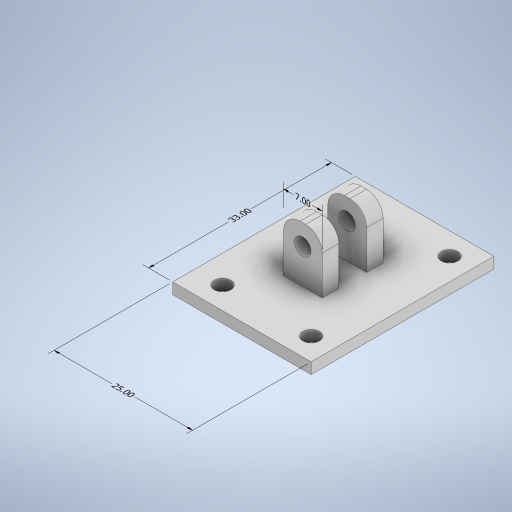
# Autodesk Inventor part: CamBracket
Saved by Autodesk Inventor 2024 (Build 280153000, 153)
## iProperties
Created: 2023-05-15
Part Number: CamBracket
Material: Generic
Document SubType Name: Modeling
Designer: User
Density: 1 g/cm^3
Appearance: Default
Author: User
Autodesk Inventor part; units mm, degrees
ref_plane "YZ Plane" through (0, 0, 0) normal (1, 0, 0) x (0, 1, 0)
ref_plane "XZ Plane" through (0, 0, 0) normal (0, 1, 0) x (-1, 0, 0)
ref_plane "XY Plane" through (0, 0, 0) normal (0, 0, 1) x (1, 0, 0)
sketch "Sketch3" plane through (0, 0, 0) normal (0, 1, 0) x (-1, 0, 0)
  line L0 (0, 0) -> (25, 0)
  line L1 (25, 0) -> (25, -33)
  line L2 (25, -33) -> (0, -33)
  line L3 (0, -33) -> (0, 0)
  dimension "d6" = 25
  dimension "d7" = 33
  constraints: 8 end point, 2 parallel, 1 horizontal, 1 perpendicular
  measures "d6" distance of L1.end L2.end
  measures "d7" distance of L0.end L1.end
extrude "Extrusion2" add sketch "Sketch3" along normal blind 2
sketch "Sketch4" plane through (0, 2, 0) normal (0, 1, 0) x (1, 0, 0)
  circle A0 centre (-4, 4) radius 1.5
  line L0 (0, 0) -> (0, 33) projected
  line L1 (-25, 0) -> (0, 0) projected
  circle A1 centre (-4, 29) radius 1.5
  line L2 (0, 33) -> (-25, 33) projected
  circle A2 centre (-20, 4) radius 1.5
  line L3 (-25, 33) -> (-25, 0) projected
  circle A3 centre (-20, 29) radius 1.5
  dimension "d16" = 3
  dimension "d17" = 4
  dimension "d18" = 4
  dimension "d19" = 3
  dimension "d20" = 4
  dimension "d21" = 4
  dimension "d22" = 3
  dimension "d23" = 16
  dimension "d24" = 4
  dimension "d25" = 5
  dimension "d26" = 3
  dimension "d27" = 4
  dimension "d28" = 16
  dimension "d29" = 25
  constraints: 4 centre point
  measures "d16" diameter of A0
  measures "d17" distance from line of L0 A0.centre
  measures "d18" distance from line of L1 A0.centre
  measures "d19" diameter of A1
  measures "d20" distance from line of L0 A1.centre
  measures "d21" distance from line of L2 A1.centre
  measures "d22" diameter of A2
  measures "d23" distance of A0.centre A2.centre
  measures "d24" distance from line of L1 A2.centre
  measures "d25" distance from line of L3 A2.centre
  measures "d26" diameter of A3
  measures "d27" distance from line of L2 A3.centre
  measures "d28" distance of A1.centre A3.centre
  measures "d29" distance of A1.centre A0.centre
extrude "Extrusion3" cut sketch "Sketch4" against normal blind 2 contours A0 | A1 | A2 | A3
sketch "Sketch5" plane through (0, 2, 0) normal (0, 1, 0) x (1, 0, 0)
  line L0 (-16, 11) -> (-9, 11)
  line L1 (-9, 11) -> (-9, 14)
  line L2 (-9, 14) -> (-16, 14)
  line L3 (-16, 14) -> (-16, 11)
  line L4 (-25, 33) -> (-25, 0) projected
  line L5 (0, 0) -> (0, 33) projected
  line L6 (-25, 0) -> (0, 0) projected
  line L7 (0, 33) -> (-25, 33) projected
  circle A0 centre (-4, 29) radius 1.5 projected
  circle A1 centre (-20, 29) radius 1.5 projected
  circle A2 centre (-4, 4) radius 1.5 projected
  circle A3 centre (-20, 4) radius 1.5 projected
  line L8 (0, 33) -> (-25, 33) projected
  line L9 (-25, 33) -> (-25, 0) projected
  line L10 (-25, 0) -> (0, 0) projected
  line L11 (0, 0) -> (0, 33) projected
  line L12 (-16, 19) -> (-9, 19)
  line L13 (-9, 19) -> (-9, 22)
  line L14 (-9, 22) -> (-16, 22)
  line L15 (-16, 22) -> (-16, 19)
  dimension "d32" = 7
  dimension "d36" = 11
  dimension "d37" = 3
  dimension "d39" = 7
  dimension "d40" = 3
  dimension "d41" = 11
  dimension "d42" = 9
  dimension "d43" = 9
  constraints: 16 end point, 4 parallel, 2 horizontal, 2 perpendicular
  measures "d32" distance of L0.start L0.end
  measures "d36" distance between parallel lines of L6 L0
  measures "d37" distance of L2.end L0.start
  measures "d39" distance of L14.end L13.end
  measures "d40" distance of L13.end L12.end
  measures "d41" distance between parallel lines of L8 L14
  measures "d42" distance between parallel lines of L4 L3
  measures "d43" distance between parallel lines of L4 L15
extrude "Extrusion4" add sketch "Sketch5" along normal blind 10 contours L3 L2 L1 L0 | L15 L14 L13 L12
sketch "Sketch6" plane through (-16, 2, -11) normal (0, 0, 1) x (1, 0, 0)
  circle A0 centre (3.5, 6.2876) radius 1.5
  line L0 (0, 0) -> (0, 10) projected
  line L1 (7, 0) -> (7, 10) projected
  point P0 (16, -2)
  dimension "d46" = 3
  dimension "d47" = 3.5
  dimension "d51" = 3.5
  constraints: 1 centre point
  measures "d46" diameter of A0
  measures "d47" distance from line of L0 A0.centre
  measures "d51" distance from line of L1 A0.centre
extrude "Extrusion5" cut sketch "Sketch6" against normal blind 13.5
fillet "Fillet1" radius 3 4 edges at (-9, 12, -20.5) (-9, 12, -12.5) (-16, 12, -12.5) (-16, 12, -20.5)
body "Solid2"
